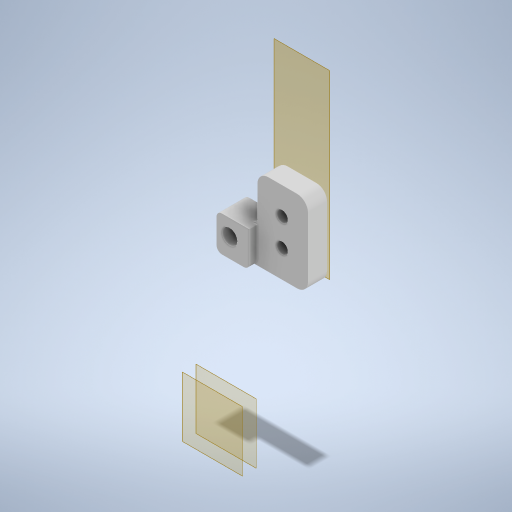
# Autodesk Inventor part: base-tensioner
Saved by Autodesk Inventor 2024 (Build 280153000, 153)
## iProperties
Created: 2024-03-17
Part Number: base-tensioner
Material: Generic
Document SubType Name: Modeling
Designer: MaartenGeorgesBuelen
Density: 1 g/cm^3
Appearance: Default
Author: MaartenGeorgesBuelen
## iProperties of the stored document base-tensioner_3DPrint.ipt
Created: 2024-03-21
Part Number: base-tensioner_3DPrint
Material: Generic
Document SubType Name: Modeling
Designer: MaartenGeorgesBuelen
Density: 1 g/cm^3
Appearance: Default
Author: MaartenGeorgesBuelen
Autodesk Inventor part; units mm, degrees
note: some values were not read from the file. Chosen so that the rebuilt part matches the saved one: edges of "Fillet10".
ref_plane "YZ Plane" through (0, 0, 0) normal (1, 0, 0) x (0, 1, 0)
ref_plane "XZ Plane" through (0, 0, 0) normal (0, 1, 0) x (-1, 0, 0)
ref_plane "XY Plane" through (0, 0, 0) normal (0, 0, 1) x (1, 0, 0)
ref_plane "Work Plane1" through (0, 0, 0) normal (0, 0, 1) x (1, 0, 0)
ref_plane "Work Plane2" through (0, 0, 0) normal (0, 0, 1) x (1, 0, 0)
sketch "Sketch6" plane through (0, 0, 0) normal (0, 0, 1) x (1, 0, 0)
  line L0 (20, 33.25) -> (1.5, 33.25) projected
  line L1 (20, 33.25) -> (20, 108.5) projected
  line L2 (1.5, 108.5) -> (20, 108.5) projected
  line L3 (1.5, 33.25) -> (1.5, 44.75) projected
  circle A0 centre (10.5, 63.5) radius 2.1 projected
  circle A1 centre (10.5, 53.5) radius 2.1 projected
  line L4 (20, 73.5) -> (-19.5, 73.5)
  line L5 (-19.5, 73.5) -> (-19.5, 43.5)
  line L6 (-19.5, 43.5) -> (20, 43.5)
  line L7 (20, 43.5) -> (20, 73.5)
  line L8 (-71.5, 45.5) -> (-71.5, 108.5) projected
  line L9 (-19.5, 73.5) -> (1.5, 73.5)
  line L10 (1.5, 73.5) -> (1.5, 56.5)
  line L11 (1.5, 56.5) -> (-19.5, 56.5)
  line L12 (-19.5, 56.5) -> (-19.5, 73.5)
  line L13 (-10.5, 43.5) -> (-19.5, 43.5)
  line L14 (-19.5, 43.5) -> (-19.5, 56.5)
  line L15 (-19.5, 56.5) -> (-10.5, 56.5)
  line L16 (-10.5, 56.5) -> (-10.5, 43.5)
  line L17 (4.5, 44.75) -> (1.5, 44.75) projected
  line L18 (1.5, 56.25) -> (1.5, 108.5) projected
  line L19 (1.5, 56.25) -> (4.5, 56.25) projected
  line L20 (4.5, 56.25) -> (4.5, 44.75) projected
  point P0 (0, 0)
  point P1 (20, 43.5)
  point P2 (-71.5, 60.5)
  point P3 (1.5, 73.5)
  point P4 (1.5, 43.5)
  point P5 (1.5, 73.5)
  point P6 (1.5, 73.5)
  dimension "d28" = 10
  dimension "d29" = 10
  dimension "d92" = 30
  dimension "d94" = 17
  dimension "d95" = 9
  constraints: 24 end point, 6 parallel, 3 horizontal, 3 perpendicular, 3 point on line
  measures "d28" distance from line of L4 A0.centre
  measures "d29" distance from line of L6 A1.centre
  measures "d92" distance from line of A0.centre L5
  measures "d94" distance of L9.end L10.end
  measures "d95" distance between parallel lines of L16 L14
extrude "Extrusion5" add sketch "Sketch6" along normal blind 7 contours L6 L3 L17 L20 L19 L18 L10 L4 L1 | L6 L16 L11 L18 L19 L20 L17 L3
ref_plane "Work Plane3" through (0, 0, 22) normal (0, 0, 1) x (1, 0, 0)
ref_plane "Work Plane4" through (0, 0, 17) normal (0, 0, 1) x (1, 0, 0)
sketch "Sketch17" plane through (0, 0, 17) normal (0, 0, 1) x (1, 0, 0)
  line L0 (-13, 58.5) -> (0, 58.5) projected
  line L1 (0, 58.5) -> (0, 88.5) projected
  line L2 (0, 88.5) -> (-13, 88.5) projected
  line L3 (-13, 88.5) -> (-13, 58.5) projected
  circle A0 centre (-5.7, 50.5) radius 2.8
  line L4 (1.5, 56.5) -> (-10.5, 56.5) projected
  line L5 (20, 43.5) -> (20, 73.5) projected
  line L6 (20, 73.5) -> (1.5, 73.5) projected
  line L7 (-10.5, 43.5) -> (20, 43.5) projected
  line L8 (-10.5, 56.5) -> (-10.5, 43.5) projected
  line L9 (1.5, 73.5) -> (1.5, 56.5) projected
  line L10 (1.5, 56.5) -> (-10.5, 56.5) projected
  point P0 (0, 0)
  point P1 (-6.5, 58.5)
  dimension "d75" = 7.3
  dimension "d88" = 5.6
  dimension "d103" = 7
  constraints: 1 centre point, 1 midpoint
  measures "d75" distance from line of L3 A0.centre
  measures "d88" diameter of A0
  measures "d103" distance from line of L7 A0.centre
extrude "Extrusion16" cut sketch "Sketch17" against normal through all contours A0
fillet "Fillet8" radius 4 3 edges at (20, 73.5, 3.5) (20, 43.5, 3.5) (1.5, 73.5, 3.5)
sketch "Sketch19" plane through (0, 0, 7) normal (0, 0, 1) x (1, 0, 0)
  line L0 (20, 47.5) -> (20, 69.5) projected
  line L1 (16, 73.5) -> (5.5, 73.5) projected
  line L2 (-10.5, 43.5) -> (16, 43.5) projected
  line L3 (-10.5, 43.5) -> (16, 43.5) projected
  line L4 (-10.5, 56.5) -> (1.5, 56.5)
  line L5 (1.5, 56.5) -> (1.5, 43.5)
  line L6 (1.5, 43.5) -> (-10.5, 43.5)
  line L7 (-10.5, 43.5) -> (-10.5, 56.5)
  circle A0 centre (-5.7, 50.5) radius 2.8 projected
  arc A1 (16, 43.5) -> (20, 47.5) centre (16, 47.5) ccw projected
  arc A2 (20, 69.5) -> (16, 73.5) centre (16, 69.5) ccw projected
  line L8 (1.5, 69.5) -> (1.5, 56.5) projected
  line L9 (1.5, 56.5) -> (-10.5, 56.5) projected
  line L10 (-10.5, 56.5) -> (-10.5, 43.5) projected
  arc A3 (5.5, 73.5) -> (1.5, 69.5) centre (5.5, 69.5) ccw projected
  point P0 (0, 0)
  point P1 (1.5, 43.5)
  point P2 (-15.5, 43.5)
  dimension "d99" = 18.5
  constraints: 8 end point, 2 parallel, 1 horizontal, 1 perpendicular, 1 point on line
  measures "d99" distance between parallel lines of L0 L5
extrude "Extrusion18" add sketch "Sketch19" along normal blind 3 contours L2 L7 L4 L5
fillet "Fillet10" radius 2 4 edges at (-10.5, 56.5, 5) (1.5, 43.5, 8.5) (-10.5, 43.5, 5) (1.5, 56.5, 3.5)
body "Solid2"
